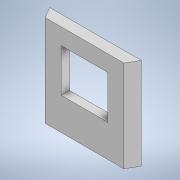
# Autodesk Inventor part: SatelliteSideWallSensor_v2
Saved by Autodesk Inventor 2020 (Build 240168000, 168)
## iProperties
Created: 2020-03-05
Part Number: SatelliteSideWallSensor_v2
Material: Generic
Document SubType Name: Modeling
Designer: WANG
Density: 1 g/cm^3
Appearance: Default
Author: WANG
Autodesk Inventor part; units mm, degrees
ref_plane "YZ Plane" through (0, 0, 0) normal (1, 0, 0) x (0, 1, 0)
ref_plane "XZ Plane" through (0, 0, 0) normal (0, 1, 0) x (-1, 0, 0)
ref_plane "XY Plane" through (0, 0, 0) normal (0, 0, 1) x (1, 0, 0)
sketch "Sketch1" plane through (0, 0, 0) normal (0, 1, 0) x (-1, 0, 0)
  line L0 (-107.95, -0.0035) -> (-53.978, 93.4857)
  line L1 (-53.978, 93.4857) -> (53.972, 93.4892)
  line L2 (53.972, 93.4892) -> (107.95, 0.0035)
  line L3 (107.95, 0.0035) -> (53.978, -93.4857)
  line L4 (53.978, -93.4857) -> (-53.972, -93.4892)
  line L5 (-53.972, -93.4892) -> (-107.95, -0.0035)
  line L6 (-92.964, 0.0336) -> (-46.4529, 80.526)
  line L7 (-46.4529, 80.526) -> (46.5111, 80.4924)
  line L8 (46.5111, 80.4924) -> (92.964, -0.0336)
  line L9 (92.964, -0.0336) -> (46.4529, -80.526)
  line L10 (46.4529, -80.526) -> (-46.5111, -80.4924)
  line L11 (-46.5111, -80.4924) -> (-92.964, 0.0336)
  line L12 (53.978, -93.4857) -> (46.4529, -80.526)
  line L13 (-53.972, -93.4892) -> (-46.5111, -80.4924)
  point P0 (0, 0)
  point P1 (0, 0)
  point P2 (0, 0)
  point P3 (0, 0)
  dimension "d0" = 215.9
  dimension "d1" = 14.986
  constraints: 28 end point, 2 coincident, 26 other
  measures "d0" distance of L0.start L2.end
  measures "d1" distance of L0.start L6.start
extrude "Extrusion1" add sketch "Sketch1" along normal blind 107.95 contours L13 L10 L12 L4
sketch "Sketch2" plane through (46.5111, 0, -80.4924) normal (-0.0003616, 0, 0.9999999) x (0.9999999, 0, 0.0003616)
  line L0 (-92.9641, 0) -> (-92.9641, 107.95) projected
  line L1 (-92.9641, 107.95) -> (0, 107.95) projected
  line L2 (-92.9641, 0) -> (0, 0) projected
  line L3 (0, 0) -> (0, 107.95) projected
  line L4 (-73.9141, 88.9) -> (-19.05, 88.9)
  line L5 (-19.05, 88.9) -> (-19.05, 38.1)
  line L6 (-19.05, 38.1) -> (-73.9141, 38.1)
  line L7 (-73.9141, 38.1) -> (-73.9141, 88.9)
  point P0 (-46.482, 0)
  dimension "d4" = 19.05
  dimension "d5" = 19.05
  dimension "d6" = 38.1
  dimension "d7" = 19.05
  constraints: 8 end point, 2 parallel, 1 horizontal, 1 perpendicular
  measures "d4" distance from line of L0 L4.start
  measures "d5" distance from line of L1 L4.start
  measures "d6" distance from line of L2 L5.end
  measures "d7" distance from line of L3 L5.end
extrude "Extrusion2" cut sketch "Sketch2" against normal up to surface (12.9965 mm away) contours L4 L5 L6 L7
sketch "Sketch3" plane through (53.972, 0, -93.4892) normal (-0.000032, 0, -1) x (-1, 0, 0.000032)
  line L0 (0, 107.95) -> (107.95, 107.95) projected
  line L1 (0, 0) -> (0, 107.95) projected
  line L2 (26.5062, 88.9) -> (81.3702, 88.9) projected
  line L3 (26.5062, 38.1) -> (26.5062, 88.9) projected
  line L4 (81.3702, 88.9) -> (81.3702, 38.1) projected
  line L5 (81.3702, 38.1) -> (26.5062, 38.1) projected
  line L6 (20.1562, 95.25) -> (87.7202, 95.25)
  line L7 (87.7202, 95.25) -> (87.7202, 31.75)
  line L8 (87.7202, 31.75) -> (20.1562, 31.75)
  line L9 (20.1562, 31.75) -> (20.1562, 95.25)
  point P0 (53.975, 0)
  dimension "d12" = 6.35
  dimension "d13" = 6.35
  dimension "d14" = 6.35
  dimension "d15" = 6.35
  constraints: 8 end point, 2 parallel, 1 horizontal, 1 perpendicular
  measures "d12" distance from line of L2 L6.start
  measures "d13" distance from line of L3 L6.start
  measures "d14" distance from line of L4 L7.end
  measures "d15" distance from line of L5 L7.end
extrude "Extrusion3" cut sketch "Sketch3" against normal blind 3.175 contours L2 L4 L5 L3 | L6 L7 L8 L9
equation "\"d7\" = d4"
equation "\"d14\" = d13"
equation "\"d15\" = d12"
body "Solid1"
